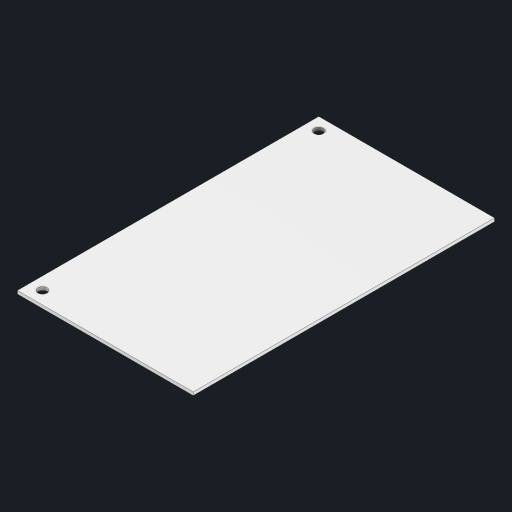
# Autodesk Inventor part: shoot2
Saved by Autodesk Inventor 2023 (Build 270158000, 158)
## iProperties
Created: 2023-04-09
Part Number: shoot2
Material: ABS Plastic
Document SubType Name: Modeling
Designer: Windows Macbook
Density: 1.06 g/cm^3
Appearance: Smooth - White
Author: Windows Macbook
Autodesk Inventor part; units mm, degrees
ref_plane "YZ Plane" through (0, 0, 0) normal (1, 0, 0) x (0, 1, 0)
ref_plane "XZ Plane" through (0, 0, 0) normal (0, 1, 0) x (-1, 0, 0)
ref_plane "XY Plane" through (0, 0, 0) normal (0, 0, 1) x (1, 0, 0)
sketch "Sketch1" plane through (0, 0, 0) normal (0, 1, 0) x (-1, 0, 0)
  line L0 (0, 0) -> (0, -152.4)
  line L1 (0, -152.4) -> (88.9, -152.4)
  line L2 (88.9, -152.4) -> (88.9, 0)
  line L3 (88.9, 0) -> (0, 0)
  dimension "d0" = 152.4
  dimension "d1" = 88.9
  constraints: 8 end point, 3 perpendicular, 1 vertical
  measures "d0" distance of L0.start L0.end
  measures "d1" distance of L0.end L1.end
extrude "Extrusion1" add sketch "Sketch1" along normal blind 1.5875
sketch "Sketch2" plane through (0, 1.5875, 0) normal (0, 1, 0) x (1, 0, 0)
  line L0 (-88.9, 0) -> (0, 0) projected
  line L1 (-88.9, 0) -> (-88.9, 12.7)
  line L2 (-88.9, 152.4) -> (-88.9, 0) projected
  line L3 (-88.9, 12.7) -> (-76.2, 0)
  line L4 (-76.2, 0) -> (-88.9, 0)
  line L5 (-88.9, 0) -> (-82.55, 6.35)
  line L6 (0, 0) -> (0, 12.7)
  line L7 (0, 0) -> (0, 152.4) projected
  line L8 (-88.9, 152.4) -> (-76.2, 152.4)
  line L9 (0, 152.4) -> (-88.9, 152.4) projected
  line L10 (-76.2, 152.4) -> (-88.9, 139.7)
  line L11 (-88.9, 139.7) -> (-88.9, 152.4)
  line L12 (-88.9, 152.4) -> (-82.55, 146.05)
  line L13 (-88.9, 152.4) -> (-79.9197, 152.4) construction
  dimension "d4" = 12.7
  dimension "d5" = 45
  dimension "d6" = 12.7
  dimension "d14" = 12.7
  dimension "d15" = 45
  dimension "d16" = 45
  constraints: 20 end point, 4 point on line, 2 coincident, 2 midpoint, 2 perpendicular, 1 equal length, 1 horizontal
  measures "d4" distance of L0.start L1.end
  measures "d5" angle of L1 L3
  measures "d6" distance of L0.end L6.end
  measures "d14" distance of L2.start L8.end
  measures "d15" angle of L8 L10
  measures "d16" angle of L12 L13
hole "Hole1" at (-82.55, 1.5875, -6.35) at (-82.55, 1.5875, -146.05) direction (0, -1, 0) diameter 4.7625 end through all
body "Solid1"
